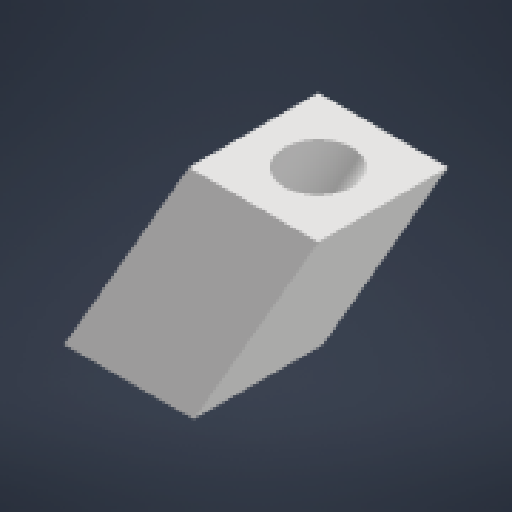
# Autodesk Inventor part: TestSoporte
Saved by Autodesk Inventor 2026.1 (Build 301233000, 233)
## iProperties
Created: 2025-10-11
Part Number: TestSoporte
Material: Generic
Document SubType Name: Modeling
Designer: tito.luyo
Density: 1 g/cm^3
Appearance: Default
soporte_largo: 15.000 mm
soporte_ancho: 15.000 mm
soporte_hueco_diametro: 7.900 mm
soporte_hueco_pos_ancho: 7.500 mm
soporte_hueco_pos_largo: 7.500 mm
soporte_inclinacion: 60.00 deg
soporte_alterura: 25.000 mm
d7: 0.00 deg
d8: 0.00 deg
tol1: 0.100 mm
tol2: 0.200 mm
tol3: 0.300 mm
tol4: 0.400 mm
tol5: 0.500 mm
tol6: 0.600 mm
tol7: 0.700 mm
tol8: 0.800 mm
tol9: 0.900 mm
tol: 7.000 mm
Author: tito.luyo
Autodesk Inventor part; units mm, degrees
ref_plane "YZ Plane" through (0, 0, 0) normal (1, 0, 0) x (0, 1, 0)
ref_plane "XZ Plane" through (0, 0, 0) normal (0, 1, 0) x (-1, 0, 0)
ref_plane "XY Plane" through (0, 0, 0) normal (0, 0, 1) x (1, 0, 0)
sketch "Sketch1" plane through (0, 0, 0) normal (0, 1, 0) x (-1, 0, 0)
  line L0 (0, 0) -> (15, 0)
  line L1 (15, 0) -> (15, -15)
  line L2 (15, -15) -> (0, -15)
  line L3 (0, -15) -> (0, 0)
  circle A0 centre (7.5, -7.5) radius 3.95
  dimension "soporte_largo" = 15
  dimension "soporte_ancho" = 15
  dimension "soporte_hueco_diametro" = 7.9
  dimension "soporte_hueco_pos_ancho" = 7.5
  dimension "soporte_hueco_pos_largo" = 7.5
  constraints: 8 end point, 2 parallel, 1 centre point, 1 horizontal, 1 perpendicular
  measures "soporte_largo" distance of L1.end L2.end
  measures "soporte_ancho" distance of L0.end L1.end
  measures "soporte_hueco_diametro" diameter of A0
  measures "soporte_hueco_pos_ancho" distance from line of L2 A0.centre
  measures "soporte_hueco_pos_largo" distance from line of L1 A0.centre
sketch "Sketch2" plane through (0, 0, 0) normal (0, 0, 1) x (1, 0, 0)
  line L0 (0, 0) -> (14.4338, 25)
  line L1 (0, 0) -> (28.8675, 0) construction
  dimension "soporte_inclinacion" = 60
  dimension "soporte_alterura" = 25
  constraints: 4 end point, 1 equal length, 1 horizontal
  measures "soporte_inclinacion" angle of L1 L0
  measures "soporte_alterura" distance from line of L0.end L1
sweep "Sweep1" add profiles "Sketch1" path "Sketch2"
equation "\"soporte_hueco_pos_ancho\" = 0.5 * soporte_ancho"
equation "\"soporte_hueco_pos_largo\" = 0.5 * soporte_largo"
equation "\"tol1\" = 0.1"
equation "\"tol2\" = 0.2"
equation "\"tol3\" = 0.3"
equation "\"tol4\" = 0.4"
equation "\"tol5\" = 0.5"
equation "\"tol6\" = 0.6"
equation "\"tol7\" = 0.7"
equation "\"tol8\" = 0.8"
equation "\"tol9\" = 0.9"
equation "\"tol\" = 7"
